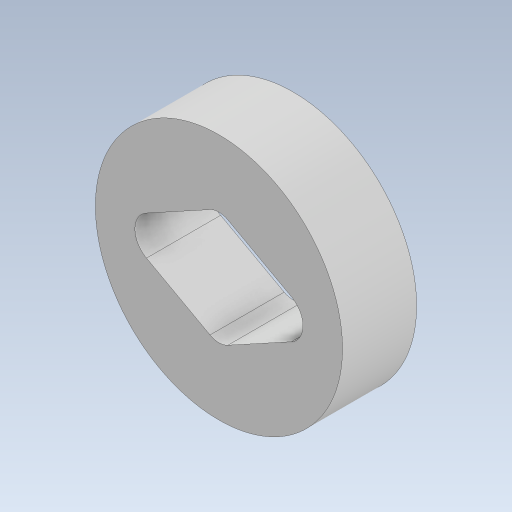
# Autodesk Inventor part: 零件14
Saved by Autodesk Inventor 2023 (Build 270158000, 158)
## iProperties
Created: 2023-04-16
Part Number: 零件14
Material: 一般
Document SubType Name: Modeling
Designer: JOU
Density: 1 g/cm^3
Appearance: 預設
Author: JOU
Autodesk Inventor part; units mm, degrees
ref_plane "YZ Plane" through (0, 0, 0) normal (1, 0, 0) x (0, 1, 0)
ref_plane "XZ Plane" through (0, 0, 0) normal (0, 1, 0) x (-1, 0, 0)
ref_plane "XY Plane" through (0, 0, 0) normal (0, 0, 1) x (1, 0, 0)
sketch "草圖4" plane through (0, 0, 0) normal (0, 0, 1) x (1, 0, 0)
  circle A0 centre (0, 0) radius 2.1
  circle A1 centre (0, 0) radius 5
  line L0 (-2.932, 0.7895) -> (-0.36, 2.1968)
  line L1 (-0.36, -2.1968) -> (-2.932, -0.7895)
  arc A2 (-2.932, 0.7895) -> (-2.932, -0.7895) centre (-2.5, 0) ccw
  arc A3 (-0.36, -2.1968) -> (0.36, -2.1968) centre (0, -1.5389) ccw
  arc A4 (0.36, 2.1968) -> (-0.36, 2.1968) centre (0, 1.5389) ccw
  line L2 (2.932, -0.7895) -> (0.36, -2.1968)
  line L3 (0.36, 2.1968) -> (2.932, 0.7895)
  arc A5 (2.932, -0.7895) -> (2.932, 0.7895) centre (2.5, 0) ccw
  dimension "d24" = 4.2
  dimension "d25" = 10
  constraints: 8 end point, 8 point on circle, 6 centre point, 2 coincident, 13 other
  measures "d24" diameter of A0
  measures "d25" diameter of A1
extrude "擠出3" add sketch "草圖4" along normal blind 3
